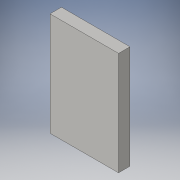
# Autodesk Inventor part: Breadboard
Saved by Autodesk Inventor 2016 (Build 200138000, 138)
## iProperties
Created: 2017-09-11
Part Number: Breadboard
Material: Generic
Document SubType Name: Modeling
Designer: student
Density: 1 g/cm^3
Appearance: Default
Author: student
Autodesk Inventor part; units mm, degrees
ref_plane "YZ Plane" through (0, 0, 0) normal (1, 0, 0) x (0, 1, 0)
ref_plane "XZ Plane" through (0, 0, 0) normal (0, 1, 0) x (-1, 0, 0)
ref_plane "XY Plane" through (0, 0, 0) normal (0, 0, 1) x (1, 0, 0)
sketch "Sketch1" plane through (0, 0, 0) normal (0, 0, 1) x (1, 0, 0)
  line L0 (-27.1018, 40.8907) -> (27.1018, 40.8907)
  line L1 (27.1018, 40.8907) -> (27.1018, -40.8973)
  line L2 (27.1018, -40.8973) -> (-27.1018, -40.8973)
  line L3 (-27.1018, -40.8973) -> (-27.1018, 40.8907)
  line L4 (-27.1018, 40.8907) -> (27.1018, -40.8973) construction
  line L5 (27.1018, 40.8907) -> (-27.1018, -40.8973) construction
  point P0 (0, -0.0033)
  constraints: 12 end point, 2 midpoint, 2 parallel, 1 horizontal, 1 perpendicular
extrude "Extrusion1" add sketch "Sketch1" along normal blind 9.0424
body "Solid1"
